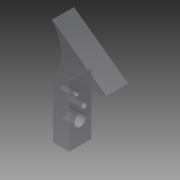
# Autodesk Inventor part: Puller Hook
Saved by Autodesk Inventor 2013 (Build 170138000, 138)
## iProperties
Created: 2013-03-21
Part Number: Puller Hook
Material: Polycarbonate, Clear
Document SubType Name: Modeling
Designer: actoennies
Mass: 9.16363 g
Surface Area: 37.3982 cm^2
Volume: 7.63636 cm^3
Density: 1.2 g/cm^3
Author: actoennies
Autodesk Inventor part; units mm, degrees
ref_plane "YZ Plane" through (0, 0, 0) normal (1, 0, 0) x (0, 1, 0)
ref_plane "XZ Plane" through (0, 0, 0) normal (0, 1, 0) x (-1, 0, 0)
ref_plane "XY Plane" through (0, 0, 0) normal (0, 0, 1) x (1, 0, 0)
sketch "Sketch1" plane through (0, 0, 0) normal (0, 0, 1) x (1, 0, 0)
  line L0 (0, 0) -> (9.525, 0)
  line L1 (9.525, 0) -> (9.525, 38.1)
  line L2 (9.525, 38.1) -> (31.75, 38.1)
  line L3 (0, 0) -> (0, 63.5) construction
  line L4 (0, 63.5) -> (-3.175, 63.5) construction
  line L5 (-3.175, 63.5) -> (31.75, 38.1)
  line L6 (0, 0) -> (0, 31.75)
  line L7 (4.7625, 0) -> (4.7625, 100.076) construction
  arc A0 (0, 31.75) -> (-3.175, 63.5) centre (-18.6849, 45.9153) ccw
  dimension "d0" = 9.525
  dimension "d1" = 38.1
  dimension "d2" = 22.225
  dimension "d3" = 63.5
  dimension "d4" = 3.175
  dimension "d5" = 4.7625
  constraints: 16 end point, 3 perpendicular, 2 midpoint, 2 parallel, 2 point on circle, 1 centre point, 1 horizontal, 1 tangent
  measures "d0" distance of L0.start L0.end
  measures "d1" distance of L0.end L1.end
  measures "d2" distance of L1.end L2.end
  measures "d3" distance of L0.start L3.end
  measures "d4" distance of L3.end L4.end
  measures "d5" distance between parallel lines of L6 L7
extrude "Extrusion1" add sketch "Sketch1" along normal blind 12.7
sketch "Sketch2" plane through (9.525, 0, 0) normal (1, 0, 0) x (0, 0, -1)
  line L0 (0, 0) -> (0, 38.1) projected
  line L1 (0, 0) -> (-12.7, 0) projected
  circle A0 centre (-6.35, 12.7) radius 3.3782
  circle A1 centre (-3.9688, 19.05) radius 1.5875
  circle A2 centre (-8.7313, 26.9875) radius 1.5875
  dimension "d8" = 6.7564
  dimension "d10" = 6.35
  dimension "d11" = 12.7
  dimension "d12" = 3.175
  dimension "d13" = 3.175
  dimension "d14" = 7.9375
  dimension "d15" = 4.7625
  dimension "d16" = 3.9688
  dimension "d17" = 19.05
  constraints: 3 centre point
  measures "d8" diameter of A0
  measures "d10" distance from line of L0 A0.centre
  measures "d11" distance from line of L1 A0.centre
  measures "d12" diameter of A1
  measures "d13" diameter of A2
  measures "d14" vertical distance of A2.centre A1.centre
  measures "d15" horizontal distance of A1.centre A2.centre
  measures "d16" distance from line of L0 A1.centre
  measures "d17" distance from line of L1 A1.centre
extrude "Extrusion2" cut sketch "Sketch2" against normal blind 12.7
fillet "Fillet1" radius 3.175 1 edges at (9.525, 38.1, 6.35)
fillet "Fillet2" radius 0.3175 1 edges at (-3.175, 63.5, 6.35)
fillet "Fillet3" radius 0.3175 1 edges at (0, 31.75, 6.35)
fillet "Fillet4" radius 0.3175 1 edges at (31.75, 38.1, 6.35)
body "Solid1"
